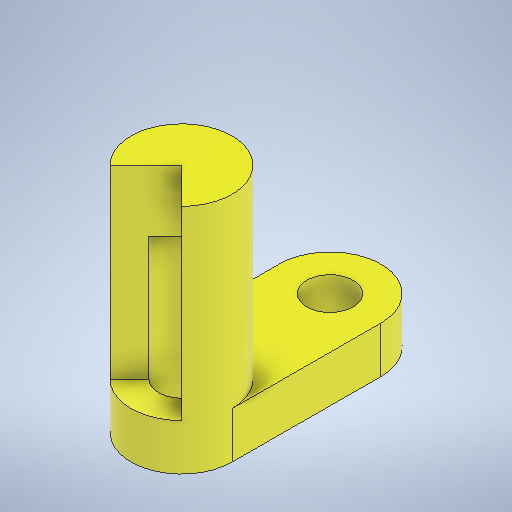
# Autodesk Inventor part: arm
Saved by Autodesk Inventor 2025.1 (Build 291241000, 241)
## iProperties
Created: 2024-10-10
Part Number: arm
Material: Generic
Document SubType Name: Modeling
Designer: m_kni
Density: 1 g/cm^3
Appearance: Default
Author: m_kni
Autodesk Inventor part; units mm, degrees
ref_plane "YZ Plane" through (0, 0, 0) normal (1, 0, 0) x (0, 1, 0)
ref_plane "XZ Plane" through (0, 0, 0) normal (0, 1, 0) x (-1, 0, 0)
ref_plane "XY Plane" through (0, 0, 0) normal (0, 0, 1) x (1, 0, 0)
sketch "Sketch1" plane through (0, 0, 0) normal (0, 1, 0) x (-1, 0, 0)
  circle A0 centre (0.0027, 10.2191) radius 5.45
  line L0 (0.0027, 10.2191) -> (0.0027, -5.7809)
  circle A1 centre (0.0027, -5.7809) radius 5.5
  circle A2 centre (0.0027, 10.2191) radius 2.5
  circle A3 centre (0.0027, -5.7809) radius 2.5
  line L1 (5.4527, 10.2191) -> (5.5026, -5.7637)
  line L2 (-5.4473, 10.2191) -> (-5.4973, -5.7637)
  point P0 (0, 0)
  point P1 (-0.0316, -5.3509)
  dimension "d0" = 10.9
  dimension "d1" = 16
  dimension "d2" = 11
  dimension "d3" = 5
  dimension "d4" = 5
  constraints: 6 end point, 4 centre point, 4 point on circle, 3 coincident, 2 tangent, 1 vertical
  measures "d0" diameter of A0
  measures "d1" distance of L0.start L0.end
  measures "d2" diameter of A1
  measures "d3" diameter of A2
  measures "d4" diameter of A3
extrude "Extrusion1" add sketch "Sketch1" along normal blind 5
sketch "Sketch2" plane through (0, 5, 0) normal (0, 1, 0) x (1, 0, 0)
  arc A0 (5.4973, 5.7637) -> (-5.5026, 5.7637) centre (-0.0027, 5.7809) ccw projected
  line L0 (-5.5026, 5.7637) -> (-5.4527, -10.2191) projected
  arc A1 (-5.4527, -10.2191) -> (5.4473, -10.2191) centre (-0.0027, -10.2191) ccw projected
  line L1 (5.4473, -10.2191) -> (5.4973, 5.7637) projected
  arc A2 (5.4973, 5.7637) -> (-5.5026, 5.7637) centre (-0.0027, 5.7809) ccw projected
  line L2 (-5.5026, 5.7637) -> (-5.4527, -10.2191) projected
  arc A3 (-5.4527, -10.2191) -> (5.4473, -10.2191) centre (-0.0027, -10.2191) ccw projected
  line L3 (5.4473, -10.2191) -> (5.4973, 5.7637) projected
  circle A4 centre (-0.0027, -10.2191) radius 2.5
  circle A5 centre (-0.0027, 5.7809) radius 2.5
  line L4 (-0.0027, -10.2191) -> (3.8511, -14.0728)
  line L5 (-0.0027, -10.2191) -> (5.4473, -10.2191) construction
  line L6 (-0.0027, -10.2191) -> (-3.8564, -14.0728)
  line L7 (-0.0027, -10.2191) -> (-0.0027, -7.7191)
  line L8 (-0.0027, -7.7191) -> (-5.1007, -12.1459)
  arc A6 (-5.4527, -10.2191) -> (5.4473, -10.2191) centre (-0.0027, -10.2191) ccw projected
  line L9 (-0.0027, -7.7191) -> (5.0953, -12.1459)
  circle A7 centre (-0.0027, -10.2191) radius 5.45
  circle A8 centre (-0.0027, -10.2191) radius 5.45
  point P0 (0, 0)
  point P1 (-3.8564, -14.0728)
  point P2 (5.0953, -12.1459)
  dimension "d7" = 5
  dimension "d8" = 5
  dimension "d9" = 45
  constraints: 12 end point, 4 coincident, 4 point on circle, 2 centre point, 1 equal length, 1 horizontal, 1 vertical, 1 vertical alignment, 6 other
  measures "d8" diameter of A5
  measures "d9" angle of L4 L5
extrude "Extrusion2" add sketch "Sketch2" along normal blind 20 contours A1 L9 A4 L8 A7 | A1 L4 A4 L9 | L8 A4 L6 A1 | L9 A4 | A4 L4 L7 L9 | L8 L7 L6 A4 | A4 L8
sketch "Sketch3" plane through (0, 0, 0) normal (0, -1, 0) x (1, 0, 0)
  arc A0 (-5.5026, -5.7637) -> (5.4973, -5.7637) centre (-0.0027, -5.7809) ccw projected
  line L0 (5.4473, 10.2191) -> (5.4973, -5.7637) projected
  arc A1 (5.4473, 10.2191) -> (-5.4527, 10.2191) centre (-0.0027, 10.2191) ccw projected
  line L1 (-5.5026, -5.7637) -> (-5.4527, 10.2191) projected
  circle A2 centre (-0.0027, -5.7809) radius 2.5
  line L2 (3.8511, 14.0728) -> (-0.0027, 10.2191) projected
  circle A3 centre (-0.0027, 10.2191) radius 2.5
  point P0 (0, 0)
  dimension "d12" = 5
  dimension "d13" = 5
  constraints: 2 centre point, 2 coincident
  measures "d12" diameter of A2
  measures "d13" diameter of A3
extrude "Extrusion3" cut sketch "Sketch3" against normal blind 4 contours A2 | A3
sketch "Sketch4" plane through (0, 5, 0) normal (0, -1, 0) x (1, 0, 0)
  circle A0 centre (-0.0027, 10.2191) radius 2.5 projected
  circle A1 centre (-0.0027, 10.2191) radius 2.5
  point P0 (0, 0)
  constraints: 1 centre point, 1 coincident, 1 concentric
extrude "Extrusion4" cut sketch "Sketch4" against normal blind 13.3375
body "Solid1"
